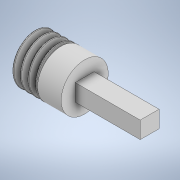
# Autodesk Inventor part: stick
Saved by Autodesk Inventor 2020 (Build 240168000, 168)
## iProperties
Created: 2020-06-07
Part Number: stick
Material: Generic
Document SubType Name: Modeling
Designer: alejandrosalazar
Density: 1 g/cm^3
Appearance: Default
Author: alejandrosalazar
Autodesk Inventor part; units mm, degrees
ref_plane "YZ Plane" through (0, 0, 0) normal (1, 0, 0) x (0, 1, 0)
ref_plane "XZ Plane" through (0, 0, 0) normal (0, 1, 0) x (-1, 0, 0)
ref_plane "XY Plane" through (0, 0, 0) normal (0, 0, 1) x (1, 0, 0)
sketch "Sketch1" plane through (0, 0, 0) normal (1, 0, 0) x (0, 1, 0)
  circle A0 centre (0, 0) radius 2.5
  dimension "d0" = 5
  constraints: 1 centre point, 1 coincident
  measures "d0" diameter of A0
extrude "Extrusion1" add sketch "Sketch1" along normal blind 5.5
thread "Thread1" size "M5x0.8" class "6g" standard "ANSI Metric M Profile" length 3
sketch "Sketch4" plane through (0, 0, 0) normal (0, 1, 0) x (0, 0, 1)
  line L0 (2.5, 0) -> (2.5, 3)
  line L1 (2.5, 3) -> (1.9068, 3)
  line L2 (1.9068, 3) -> (1.9068, 0)
  line L3 (1.9068, 0) -> (2.5, 0)
  line L4 (0, -0.6) -> (0, 3.6) projected
  constraints: 8 end point
revolve "Revolution1" cut sketch "Sketch4" angle 360 about axis through (0, 0, 0) along (1, 0, 0)
sketch "Sketch5" plane through (0, 0, 0) normal (0, 1, 0) x (0, 0, 1)
  line L0 (2.5, 0) -> (2.5, 3)
  line L1 (2.5, 3) -> (1.9068, 3)
  line L2 (1.9068, 3) -> (1.9068, 0)
  line L3 (1.9068, 0) -> (2.5, 0)
  line L4 (0, -0.6) -> (0, 3.6) projected
  constraints: 8 end point
revolve "Revolution2" add sketch "Sketch5" angle 360 about axis through (0, 0, 0) along (1, 0, 0) separate body
sketch "Sketch3" plane through (0, 0, 0) normal (0, -1, 0) x (1, 0, 0)
  line L0 (-0.4668, -1.9475) -> (-0.4001, -1.9475) construction
  line L1 (0.0666, -2.4597) -> (-0.0001, -2.5878) construction
  line L2 (-0.8001, -2.5878) -> (-0.8668, -2.4597) construction
  line L3 (-0.3334, -1.9475) -> (-0.4001, -1.8194) construction
  line L4 (-0.4001, -1.8194) -> (-0.4668, -1.9475) construction
  line L5 (-0.8001, -2.5878) -> (-0.7334, -2.4597) construction
  line L6 (-0.3334, -1.9475) -> (-0.0668, -2.4597)
  line L7 (-0.8668, -2.4597) -> (-0.7334, -2.4597) construction
  arc A0 (-0.8668, -2.4597) -> (-0.8001, -2.5002) centre (-0.8001, -2.425) ccw construction
  line L8 (0.0666, -2.4597) -> (-0.0668, -2.4597) construction
  line L9 (-0.8001, -2.5878) -> (-0.8001, -2.4597) construction
  line L10 (-0.0001, -2.5878) -> (-0.0001, -2.4597) construction
  line L11 (-0.4001, -1.8194) -> (-0.4001, -1.907) construction
  line L12 (-0.8001, -2.5002) -> (-0.0001, -2.5002)
  arc A1 (-0.8001, -2.5002) -> (-0.7334, -2.4597) centre (-0.8001, -2.425) ccw
  line L13 (-0.0668, -2.4597) -> (-0.0001, -2.5878) construction
  line L14 (-0.7334, -2.4597) -> (-0.4668, -1.9475)
  line L15 (-0.0001, -0.0002) -> (-0.0001, 0.0177)
  line L16 (-0.0001, 0.0177) -> (-0.0001, -0.0002)
  line L17 (-0.0001, -0.0002) -> (0.0334, -0.0002)
  arc A2 (-0.0668, -2.4597) -> (-0.0001, -2.5002) centre (-0.0001, -2.425) ccw
  arc A3 (-0.0001, -2.5002) -> (0.0666, -2.4597) centre (-0.0001, -2.425) ccw construction
  arc A4 (-0.4001, -1.907) -> (-0.4668, -1.9475) centre (-0.4001, -1.9822) ccw
  arc A5 (-0.3334, -1.9475) -> (-0.4001, -1.907) centre (-0.4001, -1.9822) ccw
  line L18 (-0.4001, -1.907) -> (-0.4001, -1.9475) construction
  line L19 (-0.4001, -1.9475) -> (-0.3334, -1.9475) construction
  dimension "d8" = 55
  dimension "d9" = 0.1281
  dimension "d10" = 0.1281
  dimension "Sketch3_ThreadOffset" = 0
  dimension "Sketch3_MajorRadius" = 2.5
  dimension "d13" = 0.8
  dimension "Sketch3_MinorRadius" = 1.9068
  constraints: 40 end point, 12 point on circle, 10 parallel, 8 tangent, 6 centre point, 6 collinear, 2 midpoint, 2 point on line, 1 horizontal, 1 perpendicular, 3 other
  measures "d8" angle of L6 L14
  measures "d9" distance of L3.end L0.end
  measures "d10" distance of L1.end L10.end
  measures "Sketch3_ThreadOffset" distance between parallel lines of L15 L10
  measures "Sketch3_MajorRadius" distance from line of L12 L15.start
  measures "d13" distance from line of L1.end L9
  measures "Sketch3_MinorRadius" distance edge to line of A5 L17
coil "Coil1" sketch "Sketch3" operation cut axis through (0, 0, 0) along (1, 0, 0) pitch 0.8008 turns 5.744256 hand right bodies 2
sketch "Sketch20" plane through (5.5, 0, 0) normal (1, 0, 0) x (0, 0, -1)
  line L0 (0, 0) -> (-1, 0)
  line L1 (-1, 0) -> (-1, -0.9)
  line L2 (-1, -0.9) -> (0, -0.9)
  line L3 (0, -0.9) -> (0, 0)
  line L4 (0, 0) -> (-1, 0)
  line L5 (-1, 0) -> (-1, 0.9)
  line L6 (-1, 0.9) -> (0, 0.9)
  line L7 (0, 0.9) -> (0, 0)
  line L8 (0, 0) -> (1, 0)
  line L9 (1, 0) -> (1, -0.9)
  line L10 (1, -0.9) -> (0, -0.9)
  line L11 (0, -0.9) -> (0, 0)
  line L12 (0, 0) -> (1, 0)
  line L13 (1, 0) -> (1, 0.9)
  line L14 (1, 0.9) -> (0, 0.9)
  line L15 (0, 0.9) -> (0, 0)
  point P0 (0, 0.9)
  point P1 (0, -0.9)
  dimension "d121" = 1
  dimension "d122" = 0.9
  dimension "d123" = 1
  dimension "d124" = 0.9
  dimension "d125" = 1
  dimension "d126" = 0.9
  dimension "d129" = 0.9
  constraints: 32 end point, 8 parallel, 4 horizontal, 4 perpendicular, 1 point on line
  measures "d121" distance of L2.end L1.end
  measures "d122" distance of L1.end L0.end
  measures "d123" distance of L5.end L6.end
  measures "d124" distance of L4.end L5.end
  measures "d125" distance of L9.end L10.end
  measures "d126" distance of L8.end L9.end
  measures "d129" distance of L12.end L13.end
extrude "Extrusion5" add sketch "Sketch20" along normal blind 6.9 bodies 1
equation "\"d8\" = d15"
equation "\"d9\" = 0.160083 * Sketch3_Pitch"
equation "\"d10\" = 0.160083 * Sketch3_Pitch"
equation "\"d13\" = Sketch3_Pitch"
equation "\"d15\" = 55deg"
equation "\"Sketch3_Pitch\" = 0.8"
equation "\"d38\" = 55deg"
equation "\"Sketch6_Pitch\" = 0.6"
equation "\"d64\" = 55deg"
equation "\"Sketch10_Pitch\" = 0.8"
equation "\"d85\" = 55deg"
equation "\"Sketch13_Pitch\" = 0.5"
equation "\"d106\" = 55deg"
equation "\"Sketch16_Pitch\" = 0.5"
body "Solid1"
body "Solid2"
